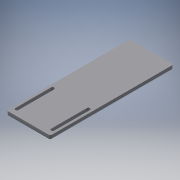
# Autodesk Inventor part: HeadBase
Saved by Autodesk Inventor 2018 (Build 220112000, 112)
## iProperties
Created: 2017-12-13
Part Number: HeadBase
Material: Generic
Document SubType Name: Modeling
Designer: reide
Density: 1 g/cm^3
Appearance: Default
Author: reide
Autodesk Inventor part; units mm, degrees
ref_plane "YZ Plane" through (0, 0, 0) normal (1, 0, 0) x (0, 1, 0)
ref_plane "XZ Plane" through (0, 0, 0) normal (0, 1, 0) x (-1, 0, 0)
ref_plane "XY Plane" through (0, 0, 0) normal (0, 0, 1) x (1, 0, 0)
sketch "Sketch1" plane through (0, 0, 0) normal (0, 0, 1) x (1, 0, 0)
  line L0 (4.8895, 31.75) -> (-4.8895, 31.75) projected
  line L1 (-4.8895, 31.75) -> (-4.8895, -31.75) projected
  line L2 (-4.8895, -31.75) -> (4.8895, -31.75) projected
  line L3 (4.8895, -31.75) -> (4.8895, 31.75) projected
  line L4 (-4.8895, -31.75) -> (-59.8895, -31.75)
  line L5 (-59.8895, -31.75) -> (-59.8895, 93.25)
  line L6 (-59.8895, 93.25) -> (-4.8895, 93.25)
  line L7 (-4.8895, 93.25) -> (-4.8895, -31.75)
  point P0 (0, 0)
  dimension "d0" = 125
  dimension "d1" = 55
  constraints: 8 end point, 2 parallel, 1 horizontal, 1 perpendicular
  measures "d0" distance of L4.end L5.end
  measures "d1" distance of L1.end L4.end
extrude "Extrusion1" add sketch "Sketch1" against normal blind 5.5 contours L1 L4 L5 L6 L7
sketch "Sketch3" plane through (-59.8895, -31.75, 0) normal (0, -1, 0) x (1, 0, 0)
  line L0 (0, 0) -> (55, 0) projected
  line L1 (0, 0) -> (0, -5.5) projected
  line L2 (55, -5.5) -> (0, -5.5) projected
  line L3 (55, 0) -> (55, -5.5) projected
  point P0 (59.8895, 0)
extrude "Extrusion2" add sketch "Sketch3" along normal blind 30
sketch "Sketch4" plane through (0, 0, -5.5) normal (0, 0, -1) x (-1, 0, 0)
  circle A0 centre (54.8895, -8.75) radius 1.25 projected
  circle A1 centre (9.8895, -8.75) radius 1.25
  circle A2 centre (54.8895, -8.75) radius 2
  circle A3 centre (9.8895, -8.75) radius 2
  line L0 (9.8895, -8.75) -> (9.8895, -53.75)
  circle A4 centre (9.8895, -53.75) radius 2
  line L1 (54.8895, -8.75) -> (54.8895, -53.75)
  circle A5 centre (54.8895, -53.75) radius 2
  line L2 (56.8895, -8.75) -> (52.8895, -8.75)
  line L3 (52.8895, -8.75) -> (52.8895, -53.75)
  line L4 (52.8895, -53.75) -> (56.8895, -53.75)
  line L5 (56.8895, -53.75) -> (56.8895, -8.75)
  line L6 (11.8895, -8.75) -> (7.8895, -8.75)
  line L7 (7.8895, -8.75) -> (7.8895, -53.75)
  line L8 (7.8895, -53.75) -> (11.8895, -53.75)
  line L9 (11.8895, -53.75) -> (11.8895, -8.75)
  point P0 (0, 0)
  dimension "d6" = 4
  dimension "d7" = 4
  dimension "d9" = 4
  dimension "d11" = 4
  dimension "d8" = 45
  dimension "d10" = 45
  constraints: 20 end point, 4 coincident, 4 horizontal alignment, 4 parallel, 2 horizontal, 2 perpendicular, 2 vertical, 1 centre point, 1 point on line, 8 other
  measures "d8" distance of L0.start L0.end
  measures "d10" distance of L1.start L1.end
extrude "Extrusion3" cut sketch "Sketch4" against normal blind 30
fillet "Fillet1" radius 2 4 edges at (-59.8895, 93.25, -2.75) (-4.8895, 93.25, -2.75) (-4.8895, -61.75, -2.75) (-59.8895, -61.75, -2.75)
fillet "Fillet2" radius 2 6 edges at (-4.8895, 15.75, -5.5) (-5.4753, 92.6642, -5.5) (-32.3895, 93.25, -5.5) (-59.3037, 92.6642, -5.5) (-59.8895, 15.75, -5.5) (-32.3895, -61.75, -5.5)
body "Solid1"
